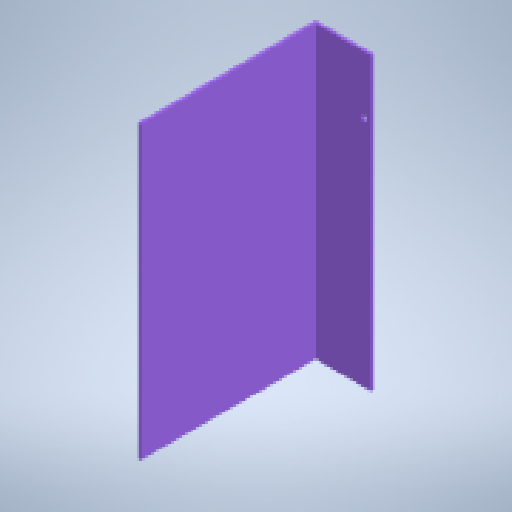
# Autodesk Inventor part: door
Saved by Autodesk Inventor 2024.3 (Build 283343010, 343A)
## iProperties
Created: 2025-11-14
Part Number: door
Material: Generic
Document SubType Name: Modeling
Designer: woyao
Density: 1 g/cm^3
Appearance: Violet
Author: woyao
Autodesk Inventor part; units mm, degrees
ref_plane "YZ Plane" through (0, 0, 0) normal (1, 0, 0) x (0, 1, 0)
ref_plane "XZ Plane" through (0, 0, 0) normal (0, 1, 0) x (-1, 0, 0)
ref_plane "XY Plane" through (0, 0, 0) normal (0, 0, 1) x (1, 0, 0)
sketch "Sketch1" plane through (0, 0, 0) normal (1, 0, 0) x (0, 1, 0)
  line L0 (0, 0) -> (500, 0)
  line L1 (500, 0) -> (500, -300)
  line L2 (500, -300) -> (0, -300)
  line L3 (0, -300) -> (0, 0)
  dimension "d0" = 300
  dimension "d1" = 500
  constraints: 8 end point, 2 parallel, 1 horizontal, 1 perpendicular
  measures "d0" distance of L0.end L1.end
  measures "d1" distance of L1.end L2.end
extrude "Extrusion1" add sketch "Sketch1" along normal blind 5
sketch "Sketch2" plane through (0, 0, -300) normal (0, 0, -1) x (-1, 0, 0)
  line L0 (0, 0) -> (-100, 0)
  line L1 (-100, 0) -> (-100, 500)
  line L2 (-100, 500) -> (0, 500)
  line L3 (0, 500) -> (0, 0)
  point P0 (-50, 0)
  dimension "d4" = 100
  dimension "d5" = 500
  constraints: 8 end point, 2 parallel, 1 horizontal, 1 midpoint, 1 perpendicular
  measures "d4" distance of L1.end L2.end
  measures "d5" distance from line of point (-50, 0) L2
extrude "Extrusion2" add sketch "Sketch2" along normal blind 5
sketch "Sketch3" plane through (0, 0, -305) normal (0, 0, -1) x (-1, 0, 0)
  circle A0 centre (-88, 400) radius 5
  line L0 (-100, 500) -> (-100, 0) projected
  line L1 (0, 500) -> (-100, 500) projected
  point P0 (0, 0)
  dimension "d8" = 10
  dimension "d9" = 12
  dimension "d10" = 100
  constraints: 1 centre point
  measures "d8" diameter of A0
  measures "d9" distance from line of L0 A0.centre
  measures "d10" distance from line of L1 A0.centre
extrude "Extrusion3" cut sketch "Sketch3" against normal blind 5
body "Solid1"
